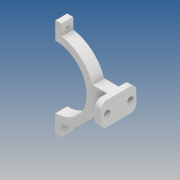
# Autodesk Inventor part: 22010_Tube End Support_V1
Saved by Autodesk Inventor 2020 (Build 240168000, 168)
## iProperties
Created: 2019-07-23
Part Number: 22010_Tube End Support_V1
Material: ABS Plastic
Document SubType Name: Modeling
Designer: MPI
Density: 1.06 g/cm^3
Appearance: Smooth - White
Author: MPI
Autodesk Inventor part; units mm, degrees
ref_plane "YZ Plane" through (0, 0, 0) normal (1, 0, 0) x (0, 1, 0)
ref_plane "XZ Plane" through (0, 0, 0) normal (0, 1, 0) x (-1, 0, 0)
ref_plane "XY Plane" through (0, 0, 0) normal (0, 0, 1) x (1, 0, 0)
sketch "Sketch1" plane through (0, 0, 0) normal (0, 1, 0) x (-1, 0, 0)
  arc A0 (0, 27) -> (0, -27) centre (0, 0) ccw
  line L0 (-49.15, 9.8171) -> (-49.15, -10.1829)
  line L1 (-49.15, -10.1829) -> (-31.3896, -10.1829)
  line L2 (-31.5059, 9.8171) -> (-49.15, 9.8171)
  arc A1 (0, 33) -> (-31.5059, 9.8171) centre (0, 0) ccw
  arc A2 (-31.3896, -10.1829) -> (0, -33) centre (0, 0) ccw
  line L3 (0, -33) -> (0, -27)
  line L4 (0, 27) -> (0, 33)
  point P0 (-41.2646, -10.1829)
  point P1 (-41.2646, 9.8171)
  point P2 (27.2866, 9.8171)
  point P3 (26.6483, -10.1829)
  dimension "d0" = 54
  dimension "d33" = 49.15
  dimension "d36" = 20
  dimension "d41" = 33
  dimension "d42" = 33
  constraints: 10 end point, 6 point on circle, 4 point on line, 3 centre point, 2 coincident, 1 horizontal, 1 parallel
  measures "d0" diameter of A0
  measures "d33" distance from line of L0 point (0, 0)
  measures "d36" distance between parallel lines of L1 L2
  measures "d41" radius of A2
  measures "d42" radius of A1
extrude "Extrusion1" add sketch "Sketch1" along normal blind 10
sketch "Sketch4" plane through (0, 10, 0) normal (0, 1, 0) x (1, 0, 0)
  line L0 (44.15, -9.8171) -> (49.15, -9.8171)
  line L1 (49.15, -9.8171) -> (49.15, 10.1829)
  line L2 (49.15, 10.1829) -> (44.15, 10.1829)
  line L3 (44.15, 10.1829) -> (44.15, -9.8171)
  line L4 (49.15, -9.8171) -> (49.15, 10.1829) projected
  line L5 (49.15, 10.1829) -> (31.3896, 10.1829) projected
  line L6 (31.5059, -9.8171) -> (49.15, -9.8171) projected
  point P0 (0, 0)
  dimension "d16" = 5
  constraints: 8 end point, 3 collinear, 2 parallel, 1 horizontal, 1 perpendicular
  measures "d16" distance of L1.end L2.end
extrude "Extrusion3" add sketch "Sketch4" along normal blind 10 and the other way blind 20
sketch "Sketch5" plane through (44.15, 10, -10.1829) normal (-1, 0, 0) x (0, 0, 1)
  circle A0 centre (10, -15) radius 2.5
  circle A1 centre (10, 5) radius 2.5
  line L0 (20, -20) -> (0, -20) projected
  line L1 (0, 10) -> (20, 10) projected
  line L2 (0, 0) -> (0, 10) projected
  line L3 (0, -20) -> (0, -10) projected
  point P0 (10.1829, -10)
  dimension "d21" = 5
  dimension "d22" = 5
  dimension "d23" = 5
  dimension "d24" = 5
  dimension "d25" = 10
  dimension "d26" = 10
  constraints: 2 centre point
  measures "d21" diameter of A0
  measures "d22" diameter of A1
  measures "d23" distance from line of A0.centre L0
  measures "d24" vertical distance of L1 A1.centre
  measures "d25" distance from line of L2 A1.centre
  measures "d26" distance from line of L3 A0.centre
extrude "Extrusion4" cut sketch "Sketch5" against normal blind 10
fillet "Fillet2" radius 5 4 edges at (46.65, -10, 9.8171) (46.65, -10, -10.1829) (46.65, 20, 9.8171) (46.65, 20, -10.1829)
sketch "Sketch7" plane through (0, 0, -33) normal (-1, 0, 0) x (0, 0, 1)
  line L0 (6, 0) -> (6, 10) projected
  line L1 (6, 10) -> (-9, 10)
  line L2 (-9, 10) -> (-9, 0)
  line L3 (-9, 0) -> (6, 0)
  line L4 (6, 0) -> (6, 10)
  line L5 (6, 10) -> (60, 10) projected
  line L6 (60, 10) -> (75, 10)
  line L7 (75, 10) -> (75, 0)
  line L8 (75, 0) -> (60, 0)
  line L9 (60, 0) -> (60, 10)
  point P0 (33, 0)
  dimension "d43" = 15
  constraints: 16 end point, 5 parallel, 2 horizontal, 2 perpendicular, 1 point on line
  measures "d43" distance of L0.end L1.end
extrude "Extrusion6" add sketch "Sketch7" against normal blind 5
sketch "Sketch8" plane through (5, 0, -33) normal (1, 0, 0) x (0, 0, 1)
  circle A0 centre (-3, -5) radius 1.65
  circle A1 centre (69, -5) radius 1.65
  line L0 (-9, 0) -> (-9, -10) projected
  line L1 (75, -10) -> (75, 0) projected
  line L2 (65.619, -10) -> (75, -10) projected
  line L3 (-9, -10) -> (0.381, -10) projected
  point P0 (33, 0)
  point P1 (-9, 10)
  point P2 (75, 10)
  point P3 (60, 10)
  point P4 (6, 10)
  dimension "d46" = 6
  dimension "d47" = 6
  dimension "d50" = 3.3
  dimension "d53" = 5
  dimension "d54" = 5
  constraints: 2 centre point, 1 equal radius, 2 other
  measures "d46" distance from line of L0 A0.centre
  measures "d47" distance from line of L1 A1.centre
  measures "d50" diameter of A0
extrude "Extrusion7" cut sketch "Sketch8" against normal blind 5
equation "\"BendRadius\" = Thickness"
equation "\"BendReliefWidth\" = Thickness"
equation "\"BendReliefDepth\" = 0.5 * Thickness"
equation "\"CornerReliefSize\" = 4 * Thickness"
equation "\"MinimumRemnant\" = 2 * Thickness"
equation "\"TransitionRadius\" = BendRadius"
equation "\"JacobiRadiusSize\" = BendRadius"
equation "\"GapSize\" = Thickness"
equation "\"Thickness\" = 0.5"
body "Solid1"
